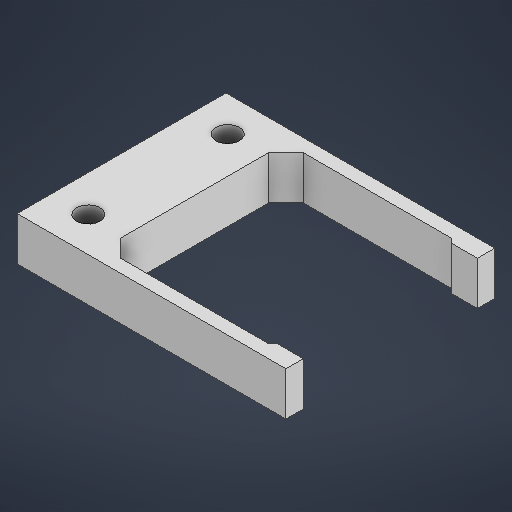
# Autodesk Inventor part: Stepper Z Mount
Saved by Autodesk Inventor 2025.1 (Build 291241000, 241)
## iProperties
Created: 2024-11-25
Part Number: Stepper Z Mount
Material: Generic
Document SubType Name: Modeling
Designer: jerem
Density: 1 g/cm^3
Appearance: Default
Author: jerem
Autodesk Inventor part; units mm, degrees
ref_plane "YZ Plane" through (0, 0, 0) normal (1, 0, 0) x (0, 1, 0)
ref_plane "XZ Plane" through (0, 0, 0) normal (0, 1, 0) x (-1, 0, 0)
ref_plane "XY Plane" through (0, 0, 0) normal (0, 0, 1) x (1, 0, 0)
sketch "Sketch1" plane through (0, 0, 0) normal (0, 1, 0) x (-1, 0, 0)
  circle A0 centre (15.5, 15.5) radius 1.5
  circle A1 centre (15.5, -15.5) radius 1.5
  circle A2 centre (-15.5, -15.5) radius 1.5
  circle A3 centre (-15.5, 15.5) radius 1.5
  circle A4 centre (0, 0) radius 11
  circle A5 centre (0, 0) radius 4
  line L0 (21, -17) -> (17, -21)
  line L1 (21, 17) -> (17, 21)
  line L2 (-17, -21) -> (-21, -17)
  line L3 (-21, 17) -> (-17, 21)
  circle A6 centre (0, 0) radius 2.5
  line L4 (17, -21) -> (-17, -21)
  line L5 (-21, -17) -> (-21, 17)
  line L6 (-17, 21) -> (17, 21)
  line L7 (21, 17) -> (21, -17)
  line L8 (0, -15.5) -> (-15.5, -15.5) construction
  line L9 (0, -15.5) -> (15.5, -15.5) construction
  line L10 (15.5, -15.5) -> (15.5, 15.5) construction
  line L11 (-15.5, -15.5) -> (-15.5, 15.5) construction
  line L12 (0, -21) -> (0, 0) construction
  line L13 (0, 0) -> (21, 0) construction
  point P0 (0, 0)
  dimension "d0" = 31
  dimension "d1" = 31
  dimension "d2" = 31
  dimension "d3" = 31
  dimension "d4" = 3
  dimension "d5" = 3
  dimension "d6" = 3
  dimension "d7" = 3
  dimension "d8" = 22
  dimension "d9" = 8
  dimension "d10" = 5
  dimension "d11" = 15.5
  dimension "d12" = 42
  dimension "d13" = 42
  dimension "d14" = 15.5
  dimension "d15" = 21
  dimension "d16" = 21
  dimension "d17" = 34
  dimension "d18" = 34
  dimension "d19" = 135
  constraints: 29 end point, 7 centre point, 6 perpendicular, 4 coincident, 3 equal length, 2 horizontal, 2 midpoint, 1 collinear, 1 vertical
  measures "d0" distance of L10.start L10.end
  measures "d1" distance of L8.end L10.start
  measures "d2" distance of L11.end L8.end
  measures "d3" distance of L10.end L11.end
  measures "d4" diameter of A0
  measures "d5" diameter of A1
  measures "d6" diameter of A2
  measures "d7" diameter of A3
  measures "d8" diameter of A4
  measures "d9" diameter of A5
  measures "d10" diameter of A6
  measures "d11" distance of L13.start L9.start
  measures "d12" distance between parallel lines of L5 L7
  measures "d13" distance between parallel lines of L6 L4
  measures "d14" distance from line of point (0, 0) L9
  measures "d15" distance of L12.start L13.start
  measures "d16" distance of L13.start L13.end
  measures "d17" distance of L7.start L7.end
  measures "d18" distance of L0.end L4.end
  measures "d19" angle of L6 L1
sketch "Sketch2" plane through (0, 0, 0) normal (0, 1, 0) x (-1, 0, 0)
  line L0 (-15.5, 15.5) -> (15.5, 15.5) construction
  line L1 (15.5, 15.5) -> (15.5, -15.5) construction
  line L2 (15.5, -15.5) -> (-15.5, -15.5) construction
  line L3 (-15.5, -15.5) -> (-15.5, 15.5) construction
  line L4 (-15.5, 15.5) -> (15.5, -15.5) construction
  line L5 (15.5, 15.5) -> (-15.5, -15.5) construction
  circle A0 centre (-15.5, -15.5) radius 1.6
  circle A1 centre (15.5, -15.5) radius 1.6
  circle A2 centre (15.5, 15.5) radius 1.6
  circle A3 centre (-15.5, 15.5) radius 1.6
  line L6 (21, -17) -> (17, -21)
  line L7 (21, -17) -> (21, 17)
  line L8 (21, 17) -> (17, 21)
  line L9 (17, 21) -> (-17, 21)
  line L10 (-17, 21) -> (-21, 17)
  line L11 (-21, 17) -> (-21, -17)
  line L12 (-21, -17) -> (-17, -21)
  line L13 (-17, -21) -> (17, -21)
  line L14 (0, -21) -> (0, -15.5) construction
  line L15 (0, 15.5) -> (0, 21) construction
  line L16 (-15.5, 0) -> (-21, 0) construction
  line L17 (15.5, 0) -> (21, 0) construction
  line L18 (-24, -24) -> (37.7656, -24)
  line L19 (37.7656, -24) -> (37.7656, 24)
  line L20 (37.7656, 24) -> (-24, 24)
  line L21 (-24, 24) -> (-24, -24)
  line L22 (-24, 20) -> (-18, 20)
  line L23 (-24, -20) -> (-18, -20)
  line L24 (-18, 20) -> (-18, 24) construction
  line L25 (-18, -20) -> (-18, -24) construction
  point P0 (0, 0)
  dimension "d20" = 31
  dimension "d22" = 3.2
  dimension "d23" = 135
  dimension "d24" = 42
  dimension "d25" = 34
  dimension "d33" = 3
  dimension "d34" = 3
  dimension "d35" = 3
  dimension "d37" = 40
  constraints: 52 end point, 12 perpendicular, 11 equal length, 10 midpoint, 8 point on line, 4 centre point, 4 coincident, 4 parallel, 3 equal radius, 2 horizontal, 1 vertical
  measures "d20" distance of L1.end L2.end
  measures "d22" diameter of A0
  measures "d23" angle of L6 L7
  measures "d24" distance between parallel lines of L9 L13
  measures "d25" distance of L6.start L7.end
  measures "d33" distance between parallel lines of L9 L20
  measures "d34" distance between parallel lines of L13 L18
  measures "d35" distance between parallel lines of L11 L21
  measures "d37" distance between parallel lines of L23 L22
sketch "Sketch3" plane through (0, 0, 0) normal (0, 1, 0) x (-1, 0, 0)
  line L0 (29.4, -16) -> (29.4, 16) construction
  circle A0 centre (29.4, -16) radius 2.7
  circle A1 centre (29.4, 16) radius 2.7
  line L1 (0, 0) -> (29.4, 0)
  dimension "d30" = 32
  dimension "d31" = 5.4
  dimension "d32" = 29.4
  constraints: 4 end point, 2 centre point, 2 coincident, 1 equal radius, 1 horizontal, 1 midpoint, 1 vertical
  measures "d30" distance of L0.start L0.end
  measures "d31" diameter of A0
  measures "d32" distance of L1.start L1.end
extrude "Extrusion1" add sketch "Sketch2" along normal blind 10 contours L7 L8 L9 L10 L22 L21 L20 L19 L18 L23 L12 L13 L6
extrude "Extrusion2" cut sketch "Sketch3" along normal through all
equation "\"d1\" = d0"
equation "\"d2\" = d0"
equation "\"d3\" = d0"
equation "\"d5\" = d4"
equation "\"d6\" = d4"
equation "\"d7\" = d4"
equation "\"d11\" = 0.5 * d0"
equation "\"d13\" = d12"
equation "\"d14\" = 0.5 * d0"
equation "\"d15\" = 0.5 * d12"
equation "\"d16\" = 0.5 * d13"
equation "\"d34\" = d33"
body "Solid1"
